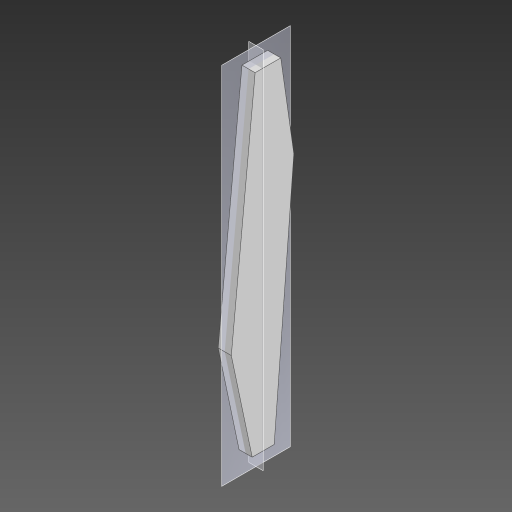
# Autodesk Inventor part: ForearmBoundingBOx
Saved by Autodesk Inventor 2023 (Build 270158000, 158)
## iProperties
Created: 2023-03-18
Part Number: ForearmBoundingBOx
Material: Generic
Document SubType Name: Modeling
Designer: Val
Density: 1 g/cm^3
Appearance: Default
Author: Val
Autodesk Inventor part; units mm, degrees
ref_plane "XZ Plane" through (0, 0, 0) normal (0, 1, 0) x (-1, 0, 0)
sketch "BoundingBox" plane through (0, 0, 0) normal (1, 0, 0) x (0, 1, 0)
  line L0 (-19.5, 16) -> (-19.5, -18)
  line L1 (-19.5, -18) -> (354.5938, -48.3648)
  line L2 (354.5938, -48.3648) -> (493.0939, -28.1898)
  line L3 (493.0939, -28.1898) -> (493.0939, 11.5)
  line L4 (493.0939, 11.5) -> (132.7202, 48.3)
  line L5 (132.7202, 48.3) -> (-19.5, 16)
  circle A0 centre (354.5938, -31.3648) radius 3.175 construction
  line L6 (354.5938, -48.3648) -> (354.5938, -31.3648) construction
  point P0 (0, 0)
  point P1 (0, 0)
  point P2 (480.5939, 0)
  point P3 (0, 0)
  point P4 (480.5939, 0)
  point P5 (60.5718, 4.3926)
  point P6 (60.5718, 4.3926)
  dimension "d0" = 19.5
  dimension "d1" = 101.98
  dimension "d2" = 18
  dimension "d3" = 16
  dimension "d4" = 12.5
  dimension "d5" = 11.5
  dimension "d6" = 48.3
  dimension "d7" = 39.6898
  dimension "d8" = 17
  dimension "d11" = 480.5939
  constraints: 14 end point, 3 coincident, 3 vertical, 1 centre point, 1 other
  measures "d0" distance from line of L0 point (0, 0)
  measures "d1" angle of L5 L0
  measures "d2" vertical distance of L0.end point (0, 0)
  measures "d3" vertical distance of L0.start point (0, 0)
  measures "d4" distance from line of L3 point (480.594, 0)
  measures "d5" vertical distance of L3.end point (480.594, 0)
  measures "d6" vertical distance of point (0, 0) L4.end
  measures "d7" distance of L2.end L3.end
  measures "d8" distance of L1.end L6.end
  measures "d11" distance of point (480.594, 0) point (0, 0)
extrude "BoundingBoxFeature" add sketch "BoundingBox" along normal mid plane 20.32
body "Solid1"
